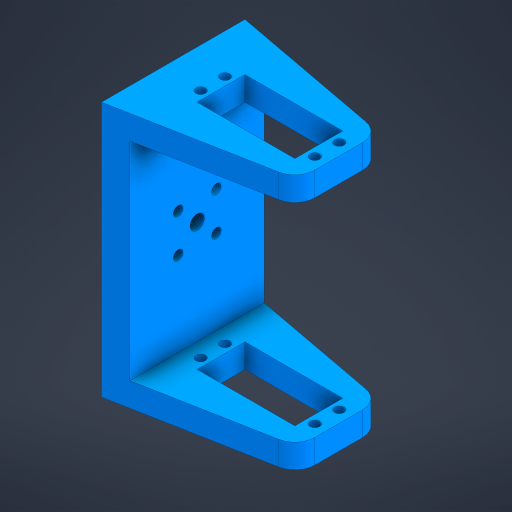
# Autodesk Inventor part: Hand-End Fork
Saved by Autodesk Inventor 2023 (Build 270158000, 158)
## iProperties
Created: 2023-08-13
Part Number: Hand-End Fork
Material: Acrylic, Clear
Document SubType Name: Modeling
Designer: Abhinav
Density: 1.19 g/cm^3
Appearance: Default(1)
Mass: 115.62 g
Surface Area: 286.493 cm^2
Volume: 97.1599 cm^3
Author: Abhinav
Autodesk Inventor part; units mm, degrees
ref_plane "YZ Plane" through (0, 0, 0) normal (1, 0, 0) x (0, 1, 0)
ref_plane "XZ Plane" through (0, 0, 0) normal (0, 1, 0) x (-1, 0, 0)
sketch "Sketch1" plane through (0, 0, 0) normal (0, 1, 0) x (-1, 0, 0)
  line L0 (20.45, 10) -> (-20.45, 10)
  line L1 (-20.45, 10) -> (-20.45, -10)
  line L2 (-20.45, -10) -> (20.45, -10)
  line L3 (20.45, -10) -> (20.45, 10)
  line L4 (20.45, 10) -> (-20.45, -10) construction
  line L5 (-20.45, 10) -> (20.45, -10) construction
  line L6 (-20.45, 10) -> (-23.9, 10)
  line L7 (-23.9, 10) -> (-23.9, 5.1) construction
  circle A0 centre (-23.9, 5.1) radius 2
  line L8 (-23.9, 5.1) -> (-20.45, 5.1) construction
  line L9 (0, 0) -> (-20.45, 0) construction
  line L10 (-20.45, -10) -> (-23.9, -10)
  line L11 (-23.9, -10) -> (-23.9, -5.1) construction
  circle A1 centre (-23.9, -5.1) radius 2
  line L12 (-23.9, -5.1) -> (-20.45, -5.1) construction
  arc A2 (-28.8, -10) -> (-21.9997, -18.2049) centre (-20.45, -10) ccw
  line L13 (-28.8, 0) -> (-28.8, -10)
  line L14 (0, 0) -> (0, -10) construction
  circle A3 centre (23.9, 5.1) radius 2
  line L15 (23.9, 5.1) -> (20.45, 5.1) construction
  circle A4 centre (23.9, -5.1) radius 2
  line L16 (23.9, -5.1) -> (20.45, -5.1) construction
  line L17 (40.45, -30) -> (-21.9997, -18.2049)
  line L18 (0, 0) -> (-20.45, 0) construction
  line L19 (30.45, 0) -> (30.45, -28.1113)
  line L20 (40.45, -28.1113) -> (40.45, 0)
  line L21 (40.45, 0) -> (40.45, -30)
  arc A5 (-21.9997, 18.2049) -> (-28.8, 10) centre (-20.45, 10) ccw
  line L22 (40.45, 30) -> (-21.9997, 18.2049)
  line L23 (30.45, 0) -> (30.45, 28.1113)
  line L24 (40.45, 28.1113) -> (40.45, 0)
  line L25 (40.45, 0) -> (40.45, 30)
  line L26 (-28.8, 10) -> (-28.8, 0)
  point P0 (20.45, 0)
  dimension "d0" = 40.9
  dimension "d1" = 20
  dimension "d2" = 3.45
  dimension "d3" = 4.9
  dimension "d4" = 4
  dimension "d10" = 10
  constraints: 54 end point, 17 symmetric about line, 6 centre point, 6 coincident, 6 point on line, 4 midpoint, 4 perpendicular, 4 point on circle, 3 parallel, 2 horizontal, 2 tangent, 1 vertical, 4 other
  measures "d0" distance of L2.end L1.end
  measures "d1" distance of L1.end L0.end
  measures "d2" distance of L0.end L6.end
  measures "d3" distance of L6.end L7.end
  measures "d4" diameter of A0
  measures "d10" distance of L20.start L19.end
extrude "Extrusion1" add sketch "Sketch1" along normal blind 10
ref_plane "Work Plane1" through (0, -43.44, 0) normal (0, -1, 0) x (1, 0, 0)
mirror "Mirror1" about plane through (0, -43.44, 0) normal (0, -1, 0) of "Extrusion1"
extrude "Extrusion2" add sketch "Sketch1" against normal blind 86.88 contours L19 L23 L22 L25 L24 L20 L21 L17
sketch "Sketch2" plane through (-30.45, -86.88, 28.1113) normal (1, 0, 0) x (0, 0, -1)
  line L0 (56.2225, 86.88) -> (56.2225, 0) projected
  line L1 (0, 0) -> (56.2225, 0)
  line L2 (56.2225, 0) -> (56.2225, 86.88)
  line L3 (56.2225, 86.88) -> (0, 86.88)
  line L4 (0, 86.88) -> (0, 0)
  line L5 (0, 86.88) -> (0, 0) construction
  line L6 (0, 0) -> (56.2225, 86.88) construction
  circle A0 centre (28.1113, 43.44) radius 3
  line L7 (20.1113, 35.44) -> (36.1113, 35.44) construction
  line L8 (36.1113, 35.44) -> (36.1113, 51.44) construction
  line L9 (36.1113, 51.44) -> (20.1113, 51.44) construction
  line L10 (20.1113, 51.44) -> (20.1113, 35.44) construction
  line L11 (20.1113, 35.44) -> (36.1113, 51.44) construction
  line L12 (36.1113, 35.44) -> (20.1113, 51.44) construction
  circle A1 centre (20.1113, 51.44) radius 2
  circle A2 centre (20.1113, 35.44) radius 2
  circle A3 centre (36.1113, 35.44) radius 2
  circle A4 centre (36.1113, 51.44) radius 2
  point P0 (28.1113, 86.88)
  dimension "d13" = 6
  dimension "d24" = 16
  dimension "d25" = 4
  constraints: 22 end point, 5 centre point, 4 coincident, 4 parallel, 3 equal radius, 3 midpoint, 3 perpendicular, 2 horizontal
  measures "d13" diameter of A0
  measures "d24" distance of L8.end L7.end
  measures "d25" diameter of A2
extrude "Extrusion3" cut sketch "Sketch2" against normal blind 10 contours A0 | A1 | A2 | A3 | A4
body "Solid1"
